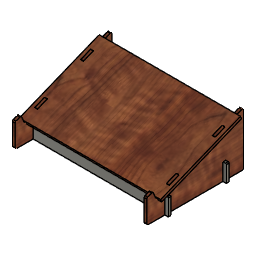
laptoptable (Autodesk Fusion 360 design; units mm, degrees)
Autodesk Fusion 360 part; units mm, degrees
sketch "Sketch1" plane through (0, 0, 0) normal (1, 0, 0) x (0, 1, 0) in component "Leg"
  line L0 (0, 0) -> (225, 0)
  line L1 (225, 0) -> (225, 125)
  line L2 (225, 125) -> (21.2612, 42.6842)
  line L3 (21.2612, 42.6842) -> (14, 60.6564)
  line L4 (14, 60.6564) -> (0, 55)
  line L5 (0, 55) -> (0, 0)
  dimension "d1" = 225
  dimension "d2" = 125
  dimension "d3" = 55
  dimension "d4" = 22
  dimension "d5" = 14
  constraint coincident L0.start L5.end
  constraint horizontal L0
  constraint perpendicular L0 L1
  constraint perpendicular L2 L3
  constraint perpendicular L0 L5
  constraint parallel L2 L4
  measures "d1" distance of L0.start L0.end
  measures "d2" distance of L0.end L1.end
  measures "d3" distance of L4.end L0.start
  measures "d4" angle of L0 L2
  measures "d5" horizontal distance of L3.end L4.end
extrude "Extrude1" add sketch "Sketch1" along normal blind 6.35 makes body 1 in component "Leg"
fillet "Fillet1" radius 3 4 edges at (3.175, 225, 125) (3.175, 21.2612, 42.6842) (3.175, 14, 60.6564) (3.175, 0, 55) on bodies 1 in component "Leg"
fillet "Fillet2" radius 3 2 edges at (3.175, 225, 0) (3.175, 0, 0) on bodies 1 in component "Leg"
sketch "Sketch1 (2)" plane through (0, -11.8419, 29.3097) normal (0, -0.374607, 0.927184) x (1, 0, 0) in component "Top"
  line L0 (0, 38.7028) -> (6.35, 38.7028)
  line L1 (6.35, 38.7028) -> (6.35, 250.9945)
  line L2 (6.35, 250.9945) -> (0, 250.9945)
  line L3 (0, 250.9945) -> (0, 38.7028)
  line L4 (14.35, 238.9945) -> (-314.35, 238.9945)
  line L5 (-314.35, 238.9945) -> (-314.35, 38.7028)
  line L6 (-314.35, 38.7028) -> (14.35, 38.7028)
  line L7 (14.35, 38.7028) -> (14.35, 238.9945)
  line L8 (-306.35, 38.7028) -> (-300, 38.7028)
  line L9 (-300, 38.7028) -> (-300, 250.9945)
  line L10 (-300, 250.9945) -> (-306.35, 250.9945)
  line L11 (-306.35, 250.9945) -> (-306.35, 38.7028)
  line L12 (0, 208.9945) -> (6.35, 208.9945)
  line L13 (0, 183.9945) -> (6.35, 183.9945)
  line L14 (-150, 238.9945) -> (-150, 38.7028) construction
  line L15 (-314.35, 138.8487) -> (14.35, 138.8487) construction
  line L16 (-300, 208.9945) -> (-306.35, 208.9945)
  line L17 (-300, 183.9945) -> (-306.35, 183.9945)
  line L18 (-300, 68.7028) -> (-306.35, 68.7028)
  line L19 (-300, 93.7028) -> (-306.35, 93.7028)
  line L20 (0, 68.7028) -> (6.35, 68.7028)
  line L21 (0, 93.7028) -> (6.35, 93.7028)
  dimension "d24" = 12
  dimension "d25" = 8
  dimension "d26" = 8
  dimension "d27" = 25
  dimension "d28" = 30
  constraint horizontal L4
  constraint vertical L5
  constraint horizontal L6
  constraint vertical L7
  constraint collinear L0 L6
  constraint coincident L3 L12.start
  constraint coincident L1 L12.end
  constraint perpendicular L1 L12
  constraint coincident L3 L13.start
  constraint coincident L1 L13.end
  constraint perpendicular L3 L13
  constraint midpoint L4 L14.start
  constraint midpoint L6 L14.end
  constraint midpoint L5 L15.start
  constraint coincident L7 L15.end
  constraint horizontal L15
  constraint symmetric L12.start L14 L16.start
  constraint symmetric L12.end L14 L16.end
  constraint symmetric L13.start L14 L17.start
  constraint symmetric L13.end L14 L17.end
  constraint symmetric L12.start L15 L20.start
  constraint symmetric L12.end L15 L20.end
  constraint symmetric L13.start L15 L21.start
  constraint symmetric L13.end L15 L21.end
  constraint symmetric L15 L16.start L18.start
  constraint symmetric L15 L16.end L18.end
  constraint symmetric L15 L17.start L19.start
  constraint symmetric L15 L17.end L19.end
  measures "d24" distance of L1.end L4
  measures "d25" distance of L1 L7
  measures "d26" distance of L5 L11
  measures "d27" distance of L12 L13
  measures "d28" distance of L4 L12
extrude "Extrude1'" add sketch "Sketch1 (2)" against normal blind 6.35 separate body contours L0 L1 L3 L6 L20 | L3 L4 L6 L9 | L1 L4 L6 L7 | L6 L8 L9 L11 L18 | L1 L3 L13 L21 | L4 L5 L6 L11 | L9 L11 L17 L19 | L1 L3 L4 L12 | L4 L9 L11 L16 makes body 2 in component "Top"
combine "Combine1" operation cut target body 1 tool bodies 2 keep tools in component "Leg"
ref_plane "WorkPlane1" through (3.175, 180, 61.7762) normal (0, 1, 0) x (0, 0, 1) in component "Support"
sketch "Sketch1 (3)" plane through (3.175, 180, 61.7762) normal (0, 1, 0) x (1, 0, 0) in component "Support"
  line L0 (-309.525, -45.0427) -> (-303.175, -45.0427)
  line L1 (-303.175, -45.0427) -> (-303.175, 61.7762)
  line L2 (-303.175, 61.7762) -> (-309.525, 61.7762)
  line L3 (-309.525, 61.7762) -> (-309.525, -45.0427)
  line L4 (-3.175, -45.0427) -> (3.175, -45.0427)
  line L5 (3.175, -45.0427) -> (3.175, 61.7762)
  line L6 (3.175, 61.7762) -> (-3.175, 61.7762)
  line L7 (-3.175, 61.7762) -> (-3.175, -45.0427)
  line L8 (11.175, 21.7762) -> (-317.525, 21.7762)
  line L9 (-317.525, 21.7762) -> (-317.525, 61.7762)
  line L10 (-317.525, 61.7762) -> (11.175, 61.7762)
  line L11 (11.175, 61.7762) -> (11.175, 21.7762)
  line L12 (-317.525, 23.8558) -> (-317.525, -51.1748)
  line L13 (11.175, -51.1748) -> (11.175, 23.8558)
  line L14 (11.175, 41.7762) -> (-317.525, 41.7762)
  dimension "d32" = 40
  constraint horizontal L8
  constraint vertical L9
  constraint horizontal L10
  constraint vertical L11
  constraint collinear L2 L10
  constraint collinear L9 L12
  constraint collinear L11 L13
  constraint midpoint L11 L14.start
  constraint midpoint L9 L14.end
  measures "d32" distance of L8 L10
extrude "Extrude1''" add sketch "Sketch1 (3)" along normal mid plane 6.35 separate body contours L3 L8 L9 L12 L14 | L1 L7 L8 L14 | L3 L9 L10 L14 | L1 L2 L3 L10 L14 | L1 L7 L10 L14 | L5 L6 L7 L10 L14 | L5 L8 L11 L13 L14 | L5 L10 L11 L14 makes body 3 in component "Support"
ref_plane "WorkPlane2" through (3.175, 112.5, 61.7762) normal (0, 1, 0) x (0, 0, 1) in component "Support"
fillet "Fillet1'" radius 2 2 edges at (14.35, 180, 40) (-314.35, 180, 40) on bodies 3 in component "Support"
fillet "Fillet2'" radius 0.5 4 edges at (-306.35, 180, 40) (-300, 180, 40) (0, 180, 40) (6.35, 180, 40) on bodies 3 in component "Support"
mirror "Mirror1" about plane through (3.175, 112.5, 61.7762) normal (0, 1, 0) of bodies 3 makes body 4 in component "Support"
combine "Combine2" operation cut target body 1 tool bodies 3 4 keep tools in component "Leg"
fillet "Fillet3" radius 0.5 4 edges at (3.175, 41.825, 0) (3.175, 48.175, 0) (3.175, 176.825, 0) (3.175, 183.175, 0) on bodies 1 in component "Leg"
fillet "Fillet4" radius 0.5 1 edges at (3.175, 24.0428, 43.808) on bodies 1 in component "Leg"
fillet "Fillet5" radius 0.5 5 edges at (3.175, 51.8583, 55.0462) (3.175, 75.0379, 64.4114) (3.175, 158.7549, 98.2352) (3.175, 181.9345, 107.6004) (3.175, 209.75, 118.8386) on bodies 1 in component "Leg"
component "Leg" placed x (1, 0, 0) y (0, 1, 0) z (0, 0, 1) at (-306.35, 0, 0)
component "Leg" placed x (1, 0, 0) y (0, 1, 0) z (0, 0, 1) at (0, 0, 0)
component "Top" placed x (1, 0, 0) y (0, 1, 0) z (0, 0, 1) at (0, 0, 0)
component "Support" placed x (1, 0, 0) y (0, 1, 0) z (0, 0, 1) at (0, 0, 0)
equation "t = 0.25 in"
equation "legwidth = 300 mm"
equation "d8 = t"
equation "d23 = legwidth"
equation "d29 = -t"
equation "d33 = t / 2"
